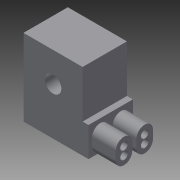
# Autodesk Inventor part: lickport_DHO_MultiFused_v0
Saved by Autodesk Inventor 2013 (Build 170138000, 138)
## iProperties
Created: 2011-06-06
Part Number: lickport_DHO_MultiFused_v0
Document SubType Name: Modeling
Designer: D Flickinger
Density: 1 g/cm^3
Material: Generic
Author: D Flickinger
Autodesk Inventor part; units mm, degrees
ref_plane "YZ Plane" through (0, 0, 0) normal (1, 0, 0) x (0, 1, 0)
ref_plane "XZ Plane" through (0, 0, 0) normal (0, 1, 0) x (-1, 0, 0)
ref_plane "XY Plane" through (0, 0, 0) normal (0, 0, 1) x (1, 0, 0)
sketch "Sketch1" plane through (0, 0, 0) normal (0, 0, 1) x (1, 0, 0)
  line L0 (-12.7, 10.16) -> (0, 10.16)
  line L1 (0, 10.16) -> (0, 0)
  line L2 (0, 0) -> (1.27, 0)
  line L3 (1.27, 0) -> (1.27, -6.35)
  line L4 (1.27, -6.35) -> (-0.0109, -6.35)
  line L5 (-0.0109, -6.35) -> (-12.7, -6.35)
  line L6 (-12.7, -6.35) -> (-12.7, 10.16)
  dimension "d0" = 12.7
  dimension "d1" = 1.27
  dimension "d2" = 6.35
  dimension "d3" = 16.51
  constraints: 14 end point, 5 parallel, 1 horizontal, 1 perpendicular
  measures "d0" distance of L0.start L0.end
  measures "d1" distance of L1.end L2.end
  measures "d2" distance of L2.end L3.end
  measures "d3" distance of L5.end L0.start
extrude "Extrusion1" add sketch "Sketch1" along normal blind 9.525
hole "Hole1" at (-6.35, 3.81, 9.525) direction (0, 0, -1) diameter 3.556 end through all
hole "Hole2" at (-12.7, -4.445, 2.54) direction (1, 0, 0) diameter 1.6002 end through all
hole "Hole3" at (-12.7, -2.667, 2.54) direction (1, 0, 0) diameter 1.6002 depth 25.4 tip angle 118
hole "Hole4" at (-12.7, -2.667, 6.985) direction (1, 0, 0) diameter 1.6002 end through all
hole "Hole5" at (-12.7, -4.445, 6.985) direction (1, 0, 0) diameter 1.6002 end through all
sketch "Sketch2" plane through (1.27, -6.35, 0) normal (1, 0, 0) x (0, 0, -1)
  circle A0 centre (-6.985, 1.905) radius 0.8001 projected
  circle A1 centre (-6.985, 3.683) radius 0.8001 projected
  circle A2 centre (-2.54, 3.683) radius 0.8001 projected
  circle A3 centre (-2.54, 1.905) radius 0.8001 projected
  arc A4 (-5.2178, 3.683) -> (-8.7522, 3.683) centre (-6.985, 3.683) ccw
  line L0 (-8.7522, 3.683) -> (-8.7522, 1.905)
  arc A5 (-8.7522, 1.905) -> (-5.2178, 1.905) centre (-6.985, 1.905) ccw
  line L1 (-5.2178, 1.905) -> (-5.2178, 3.683)
  line L2 (-4.3207, 3.683) -> (-4.3207, 1.905)
  arc A6 (-4.3207, 1.905) -> (-0.7593, 1.905) centre (-2.54, 1.905) ccw
  line L3 (-0.7593, 1.905) -> (-0.7593, 3.683)
  arc A7 (-0.7593, 3.683) -> (-4.3207, 3.683) centre (-2.54, 3.683) ccw
  constraints: 8 end point, 8 point on circle, 4 centre point
extrude "Extrusion3" add sketch "Sketch2" along normal blind 5.08
body "Solid1"
